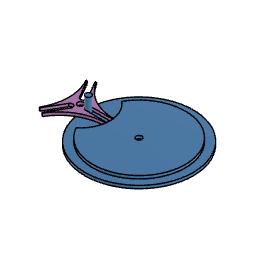
geneva mechanism v8 (Autodesk Fusion 360 design; units mm, degrees)
Autodesk Fusion 360 part; units mm, degrees
sketch "Sketch1" plane through (0, 0, 0) normal (0, 1, 0) x (1, 0, 0)
  line L0 (0, 0) -> (12.7, -21.997) construction
  line L1 (0, 0) -> (50.8, 0) construction
  line L2 (12.7, -21.997) -> (50.8, 0) construction
  circle A0 centre (0, 0) radius 25.4
  circle A1 centre (50.8, 0) radius 43.9941
  circle A2 centre (0, 0) radius 6.8059 construction
  circle A3 centre (12.7, -21.997) radius 2.54 construction
  circle A4 centre (3.403, -5.8941) radius 2.54 construction
  line L3 (1.2033, -7.1641) -> (10.5003, -23.267)
  arc A5 (10.5003, -23.267) -> (14.8997, -20.727) centre (12.7, -21.997) ccw
  line L4 (14.8997, -20.727) -> (5.6027, -4.6241)
  arc A6 (5.6027, -4.6241) -> (1.2033, -7.1641) centre (3.403, -5.8941) ccw
  line L5 (3.403, -5.8941) -> (12.7, -21.997) construction
  line L6 (10.16, -21.997) -> (10.16, 0) construction
  circle A7 centre (50.8, 0) radius 40.64
  circle A8 centre (50.8, 0) radius 40.132
  circle A9 centre (6.8059, 0) radius 2.54
  line L7 (5.6027, 4.6241) -> (14.8997, 20.727)
  line L8 (10.5003, 23.267) -> (1.2033, 7.1641)
  arc A10 (1.2033, 7.1641) -> (5.6027, 4.6241) centre (3.403, 5.8941) ccw
  circle A11 centre (-25.4, 43.9941) radius 40.64
  line L9 (-6.8059, 2.54) -> (-25.4, 2.54)
  line L10 (-25.4, -2.54) -> (-6.8059, -2.54)
  arc A12 (-6.8059, -2.54) -> (-6.8059, 2.54) centre (-6.8059, 0) ccw
  circle A13 centre (-25.4, -43.9941) radius 40.64
  circle A14 centre (0, 0) radius 2.54
  circle A15 centre (50.8, 0) radius 2.54
  circle A16 centre (50.8, 0) radius 25.4
  dimension "d1" = 25.4
  dimension "d3" = 60
  dimension "d6" = 90
  dimension "d7" = 5.08
  dimension "d10" = -0.508
  dimension "d11" = 5.08
  dimension "d13" = 360
  dimension "d14" = 5.08
  dimension "d15" = 50.8
  constraint horizontal L1
  constraint coincident L0.start L1.start
  constraint perpendicular L0 L2
  constraint coincident L0.end A0
  constraint coincident L1.end L2.end
  constraint coincident L0.end A1
  constraint concentric A0 A2
  constraint tangent A1 A2
  constraint coincident L0.end L2.start
  constraint coincident L0 A4.centre
  constraint coincident A2 A4.centre
  constraint equal A3 A4
  constraint tangent L3 A5
  constraint tangent A5 L4
  constraint parallel L3 L4
  constraint tangent L4 A6
  constraint tangent L3 A6
  constraint coincident A4.centre A6.centre
  constraint coincident A3 A5.end
  constraint coincident A3 L6.start
  constraint coincident L1 L6.end
  constraint perpendicular L1 L6
  constraint tangent A3 L6
  constraint concentric A1 A7
  constraint coincident L6.end A7
  constraint coincident A2 A9.centre
  constraint coincident A1 A9.centre
  constraint concentric A2 A14
  constraint concentric A7 A15
  constraint equal A14 A15
  constraint concentric A1 A16
  measures "d1" distance of L0.start L0.end
  measures "d3" angle of L0 L1
  measures "d6" angle of L0 L2
  measures "d7" diameter of A3
  measures "d11" diameter of A9
  measures "d14" diameter of A14
  measures "d15" diameter of A16
sketch "Sketch2" plane through (0, 0, 0) normal (0, 0, 1) x (1, 0, 0)
  circle A0 centre (-25.4, -43.9941) radius 40.64
  circle A1 centre (3.403, -5.8941) radius 2.54 construction
  line L0 (5.6027, 4.6241) -> (14.8997, 20.727)
  circle A2 centre (50.8, 0) radius 40.64
  circle A3 centre (50.8, 0) radius 2.54
  circle A4 centre (50.8, 0) radius 43.9941
  circle A5 centre (12.7, -21.997) radius 2.54 construction
  line L1 (10.5003, 23.267) -> (1.2033, 7.1641)
  line L2 (12.7, -21.997) -> (50.8, 0) construction
  circle A6 centre (50.8, 0) radius 25.4
  circle A7 centre (50.8, 0) radius 40.132
  arc A8 (5.6027, -4.6241) -> (1.2033, -7.1641) centre (3.403, -5.8941) ccw
  line L3 (0, 0) -> (12.7, -21.997) construction
  circle A9 centre (6.8059, 0) radius 2.54
  line L4 (-25.4, -2.54) -> (-6.8059, -2.54)
  arc A10 (10.5003, -23.267) -> (14.8997, -20.727) centre (12.7, -21.997) ccw
  line L5 (14.8997, -20.727) -> (5.6027, -4.6241)
  circle A11 centre (0, 0) radius 2.54
  arc A12 (-6.8059, -2.54) -> (-6.8059, 2.54) centre (-6.8059, 0) ccw
  line L6 (10.16, -21.997) -> (10.16, 0) construction
  circle A13 centre (0, 0) radius 6.8059 construction
  arc A14 (1.2033, 7.1641) -> (5.6027, 4.6241) centre (3.403, 5.8941) ccw
  line L7 (-6.8059, 2.54) -> (-25.4, 2.54)
  line L8 (3.403, -5.8941) -> (12.7, -21.997) construction
  line L9 (1.2033, -7.1641) -> (10.5003, -23.267)
  line L10 (0, 0) -> (50.8, 0) construction
  circle A15 centre (-25.4, 43.9941) radius 40.64
  circle A16 centre (0, 0) radius 25.4
  circle A17 centre (50.8, 0) radius 43.18
  dimension "d16" = -0.508
  dimension "d18" = 360
  dimension "d19" = 25.4
  dimension "d20" = 60
  dimension "d21" = 90
  dimension "d22" = 5.08
  dimension "d23" = 5.08
  dimension "d24" = 5.08
  dimension "d25" = 50.8
  dimension "d34" = 86.36
  constraint horizontal L10
  constraint coincident L3.start A11.centre
  constraint perpendicular L2 L3
  constraint coincident A5.centre A16
  constraint coincident A2.centre A3.centre
  constraint coincident A5.centre A4
  constraint concentric A13 A16
  constraint tangent A4 A13
  constraint coincident A5.centre L2.start
  constraint coincident A1.centre L3
  constraint coincident A1.centre A13
  constraint equal A1 A5
  constraint tangent A10 L9
  constraint tangent A10 L5
  constraint parallel L5 L9
  constraint tangent A8 L5
  constraint tangent A8 L9
  constraint coincident A1.centre A8.centre
  constraint coincident A10.end A5
  constraint coincident L6.start A5
  constraint coincident L6.end L10
  constraint perpendicular L6 L10
  constraint tangent A5 L6
  constraint concentric A2 A4
  constraint coincident L6.end A2
  constraint coincident A9.centre A13
  constraint coincident A9.centre A4
  constraint concentric A11 A13
  constraint concentric A2 A3
  constraint equal A3 A11
  constraint concentric A4 A6
  constraint concentric A6 A17
  measures "d19" distance of L3.start A5.centre
  measures "d20" angle of L3 L10
  measures "d21" angle of L2 L3
  measures "d22" diameter of A5
  measures "d23" diameter of A9
  measures "d24" diameter of A11
  measures "d25" diameter of A6
  measures "d34" diameter of A17
sketch "Sketch3" plane through (0, 0, 0) normal (0, 0, 1) x (1, 0, 0)
  circle A0 centre (0, 0) radius 2.54
  circle A1 centre (50.8, 0) radius 2.54
  circle A2 centre (0, 0) radius 2.54
  line L0 (0, -6.35) -> (50.8, -6.35)
  arc A3 (50.8, -6.35) -> (50.8, 6.35) centre (50.8, 0) ccw
  line L1 (50.8, 6.35) -> (0, 6.35)
  arc A4 (0, 6.35) -> (0, -6.35) centre (0, 0) ccw
  line L2 (0, 0) -> (50.8, 0) construction
  circle A5 centre (50.8, 0) radius 43.18
  point P0 (50.8, 0)
  dimension "d26" = 5.08
  dimension "d27" = 12.7
  dimension "d37" = 86.36
  constraint coincident A0.centre A2.centre
  constraint coincident P0 A1.centre
  constraint equal A1 A2
  constraint tangent L0 A3
  constraint tangent A3 L1
  constraint parallel L0 L1
  constraint tangent L1 A4
  constraint tangent L0 A4
  measures "d26" diameter of A0
  measures "d27" diameter of A3
  measures "d37" diameter of A5
extrude "Extrude1" add sketch "Sketch2" along normal blind 2.54 contours A0 L0 A4 L1 A8 A9 L4 L5 A12 A14 L7 L9 A15 A16 | A4 A9 L5 A17 | A4 A9 | A4 A9 A17 | L0 A2 A9 L5 A16 A17 | L0 A4 A9 A17 | A9 A17 makes body 1
extrude "Extrude2" add sketch "Sketch2" along normal blind 2.54 separate body contours A6 | A7 A16 picked at (23.3306, -19.7255) makes body 2
extrude "Extrude3" add sketch "Sketch2" along normal blind 12.7 separate body contours A4 A9 | A4 A9 A17 | A9 A17 makes body 3
extrude "Extrude4" add sketch "Sketch2" against normal blind 2.54 separate body contours L5 A16 A17 | A10 L5 A16 A17 | A2 A10 L5 A16 A17 | L0 A2 A9 L5 A16 A17 | A9 A17 | A2 A7 A16 | A2 A7 A16 | L0 A16 A17 | A6 | A7 A16 | A7 A16 makes body 4
extrude "Extrude5" add sketch "Sketch3" along normal blind 2.54 separate body contours L0 L1 A4 A5 makes body 5
extrude "Extrude6" add sketch "Sketch3" against normal blind 2.54 separate body contours L0 L1 A4 A5 | L0 A3 L1 A5 picked at (35.8636, 4.7103) makes body 6
move_body "Move1" bodies 1 to x (0.5, -0.866025, 0) y (0.866025, 0.5, 0) z (0, 0, 1) at (0, 0, 0)
sketch "Sketch4" plane through (0, 0, 0) normal (0, 0, 1) x (1, 0, 0)
  circle A0 centre (50.8, 0) radius 46.99
  point P0 (50.8, 0)
  dimension "d43" = 93.98
  constraint coincident P0 A0.centre
  measures "d43" diameter of A0
extrude "Extrude7" add sketch "Sketch4" against normal blind 2.54 separate body makes body 7
move_body "Move2" bodies 1 2 3 7 to x (1, 0, 0) y (0, 1, 0) z (0, 0, 1) at (0, 0, 2.54)
delete_body "RemoveBody2" bodies 4
combine "Combine1" operation cut target body 5 tool bodies 7 keep tools
copy_body "Body->Comp1" bodies 1 removing the originals makes body 8 in component "Component"
copy_body "Body->Comp2" bodies 2 removing the originals makes body 9 in component "Component'"
copy_body "Body->Comp3" bodies 3 removing the originals makes body 10 in component "Component''"
copy_body "Body->Comp4" bodies 5 removing the originals makes body 11 in component "Component'''"
copy_body "Body->Comp5" bodies 6 removing the originals makes body 12 in component "Component''''"
copy_body "Body->Comp6" bodies 7 removing the originals makes body 13 in component "Component'''''"
sketch "Sketch5" plane through (0, 0, 5.08) normal (0, 0, 1) x (-1, 0, 0)
  circle A0 centre (-50.8, 0) radius 2.54
  arc A1 (-15.8979, 19.8095) -> (-15.8979, -19.8095) centre (-50.8, 0) ccw
  arc A2 (-15.8979, 19.8095) -> (-15.8979, -19.8095) centre (0, 0) ccw
  circle A3 centre (-50.8, 0) radius 2.54
  dimension "d54" = 5.08
  constraint concentric A0 A3
  measures "d54" diameter of A3
extrude "Extrude1'" cut sketch "Sketch5" against normal through all contours A0 A3 bodies 13 in component "Component'''''"
component "Component" placed x (1, 0, 0) y (0, 1, 0) z (0, 0, 1) at (0, 0, 0)
component "Component'" placed x (1, 0, 0) y (0, 1, 0) z (0, 0, 1) at (0, 0, 0)
component "Component''" placed x (1, 0, 0) y (0, 1, 0) z (0, 0, 1) at (0, 0, 0)
component "Component'''" placed x (1, 0, 0) y (0, 1, 0) z (0, 0, 1) at (0, 0, 0)
component "Component''''" placed x (1, 0, 0) y (0, 1, 0) z (0, 0, 1) at (0, 0, 0)
component "Component'''''" placed x (1, 0, 0) y (0, 1, 0) z (0, 0, 1) at (0, 0, 0)
